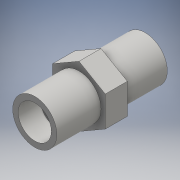
# Autodesk Inventor part: Inlet Pipe Nipple
Saved by Autodesk Inventor 2016 (Build 200138000, 138)
## iProperties
Created: 2016-12-04
Part Number: Inlet Pipe Nipple
Material: Generic
Document SubType Name: Modeling
Designer: Muhammad
Density: 1 g/cm^3
Appearance: Default
Author: Muhammad
Autodesk Inventor part; units mm, degrees
ref_plane "YZ Plane" through (0, 0, 0) normal (1, 0, 0) x (0, 1, 0)
ref_plane "XY Plane" through (0, 0, 0) normal (0, 0, 1) x (1, 0, 0)
sketch "Sketch1" plane through (0, 0, 0) normal (0, 1, 0) x (-1, 0, 0)
  line L0 (0, 0) -> (5.5, 0)
  line L1 (0, 0) -> (0, -5.5)
  line L2 (0, -5.5) -> (-4.7631, -2.75)
  line L3 (-4.7631, -2.75) -> (-4.7631, 2.75)
  line L4 (-4.7631, 2.75) -> (0, 5.5)
  line L5 (0, 5.5) -> (4.7631, 2.75)
  line L6 (4.7631, 2.75) -> (4.7631, -2.75)
  line L7 (4.7631, -2.75) -> (0, -5.5)
  dimension "d0" = 5.5
  dimension "d1" = 5.5
  constraints: 16 end point, 1 coincident, 1 horizontal, 1 vertical, 13 other
  measures "d0" distance of L0.start L0.end
  measures "d1" distance of L0.start L1.end
extrude "Extrusion1" add sketch "Sketch1" along normal mid plane 4
sketch "Sketch2" plane through (0, 0, 0) normal (0, 1, 0) x (-1, 0, 0)
  circle A0 centre (0, 0) radius 4
  dimension "d4" = 8
  constraints: 1 centre point, 1 coincident
  measures "d4" diameter of A0
extrude "Extrusion2" add sketch "Sketch2" along normal mid plane 20
sketch "Sketch3" plane through (0, 10, 0) normal (0, 1, 0) x (1, 0, 0)
  circle A0 centre (0, 0) radius 3
  dimension "d7" = 6
  constraints: 1 centre point, 1 coincident
  measures "d7" diameter of A0
hole "Hole1" at (0, 10, 0) direction (0, -1, 0) diameter 5 depth 10 tip angle 118 counterbore diameter 6 counterbore depth 4
ref_plane "Work Plane1" through (0, 0, 0) normal (0, 1, 0) x (-1, 0, 0)
mirror "Mirror1" about plane through (0, 0, 0) normal (0, 1, 0) of "Hole1"
body "Solid1"
